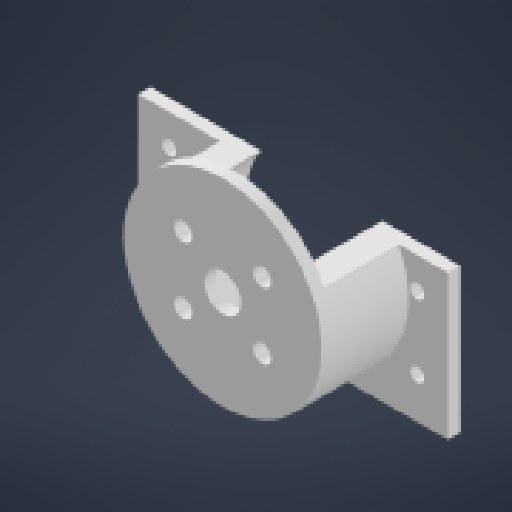
# Autodesk Inventor part: Rex Motor Bracket
Saved by Autodesk Inventor 2023 (Build 270158000, 158)
## iProperties
Created: 2022-12-08
Part Number: Rex Motor Bracket
Material: Generic
Document SubType Name: Modeling
Designer: Izack Waczko
Density: 1 g/cm^3
Appearance: Default
Author: Izack Waczko
Autodesk Inventor part; units mm, degrees
ref_plane "YZ Plane" through (0, 0, 0) normal (1, 0, 0) x (0, 1, 0)
ref_plane "XZ Plane" through (0, 0, 0) normal (0, 1, 0) x (-1, 0, 0)
sketch "Sketch1" plane through (0, 0, 0) normal (0, 0, 1) x (1, 0, 0)
  circle A0 centre (-15, 75) radius 1.7
  circle A1 centre (-15, 57.5) radius 1.7
  circle A2 centre (-75, 75) radius 1.7
  circle A3 centre (-75, 57.5) radius 1.7
  line L0 (-67.5, 62.5) -> (-67.5, 82.5)
  arc A4 (-67.5, 62.5) -> (-57.5, 52.5) centre (-57.5, 62.5) ccw
  line L1 (-32.5, 52.5) -> (-57.5, 52.5)
  arc A5 (-32.5, 52.5) -> (-22.5, 62.5) centre (-32.5, 62.5) ccw
  line L2 (-22.5, 82.5) -> (-22.5, 62.5)
  line L3 (-7.5, 82.5) -> (-22.5, 82.5)
  line L4 (-7.5, 62.5) -> (-7.5, 82.5)
  line L5 (-67.5, 82.5) -> (-82.5, 82.5)
  line L6 (-82.5, 82.5) -> (-82.5, -37.5)
  line L7 (-82.5, 52.5) -> (-57.5, 52.5)
  line L8 (-32.5, 52.5) -> (-7.5, 52.5)
  line L9 (-7.5, 52.5) -> (-7.5, 62.5)
  circle A6 centre (-41.087567, 72.129389) radius 17.98
  line L10 (-67.5, 82.5) -> (-55.775345, 82.5)
  line L11 (-22.5, 82.5) -> (-26.399789, 82.5)
  line L12 (-7.5, 52.5) -> (-82.5, 52.5)
  line L13 (-82.5, 52.5) -> (-82.5, 47.5)
  line L14 (-82.5, 47.5) -> (-7.5, 47.5)
  line L15 (-7.5, 47.5) -> (-7.5, 52.5)
  point P0 (0, 0)
  point P1 (-22.296102, 67.952867)
  dimension "d2" = 5
  constraints: 18 end point, 4 point on line, 3 perpendicular, 3 point on circle, 2 horizontal, 2 parallel, 1 other
  measures "d2" distance of L13.end L12.end
extrude "Extrusion1" add sketch "Sketch1" along normal blind 3 contours A4 L7 L6 L5 L0 | L0 L10 A6 L11 L2 A5 L1 A4 | L1 L8 L15 L14 L6 L7 | A5 L2 L3 L4 L9 L8
sketch "Sketch2" plane through (0, 0, 3) normal (0, 0, 1) x (1, 0, 0)
  circle A0 centre (-41.087567, 72.129389) radius 17.98
  line L0 (-55.775345, 82.5) -> (-82.5, 82.5)
  line L1 (-7.5, 82.5) -> (-26.399789, 82.5)
  circle A1 centre (-41.087567, 72.129389) radius 20.98
  point P0 (0, 0)
  point P1 (-59.325188, 82.5)
  point P2 (-22.849946, 82.5)
  dimension "d3" = 3
  constraints: 1 centre point
  measures "d3" radial gap between concentric circles of A0 A1
ref_plane "Work Plane1" through (-53.798179, 52.016597, 21) normal (0, 0, 1) x (0.817541, 0.5758704, 0)
extrude "Extrusion2" add sketch "Sketch2" along normal up to surface (18 mm away) contours A0 L1 A1 L0 picked at (-21.478975, 69.046328)
sketch "Sketch3" plane through (-41.087567, 72.129389, 21) normal (0, 0, 1) x (1, 0, 0)
  arc A0 (-18.237621, 10.370611) -> (18.237621, 10.370611) centre (0, 0) ccw
  circle A1 centre (0, 0) radius 4.485
  arc A2 (-14.687778, 10.370611) -> (14.687778, 10.370611) centre (0, 0) ccw construction
  line L0 (0, 0) -> (11.25, 0) construction
  line L1 (8, 0) -> (8, -8) construction
  line L2 (0, 0) -> (0, -11.25) construction
  circle A3 centre (8, -8) radius 2.2
  circle A4 centre (-8, -8) radius 2.2
  circle A5 centre (0, 0) radius 20.98
  circle A6 centre (8, 8) radius 2.2
  circle A7 centre (-8, 8) radius 2.2
  point P0 (41.087567, -72.129389)
  point P1 (18.237621, 10.370611)
  point P2 (-18.237621, 10.370611)
  dimension "d6" = 8
  dimension "d7" = 4.4
  dimension "d20" = 16
  dimension "d21" = 8
  constraints: 6 end point, 5 centre point, 3 symmetric about line, 2 coincident, 1 concentric, 1 horizontal, 1 perpendicular, 1 point on line, 1 vertical, 3 other
  measures "d6" distance of L1.start L1.end
  measures "d7" diameter of A3
  measures "d20" distance of A4.centre L1.end
  measures "d21" distance from line of L1 A0.centre
extrude "Extrusion3" add sketch "Sketch3" along normal blind 3
fillet "Fillet1" radius 5 4 edges at (-82.5, 82.5, 1.5) (-82.5, 47.5, 1.5) (-7.5, 47.5, 1.5) (-7.5, 82.5, 1.5)
fillet "Fillet2" radius 5 1 edges at (-41.0876, 51.1494, 3)
fillet "Fillet3" radius 5 1 edges at (-59.3252, 61.7588, 24)
sketch "Sketch4" plane through (0, 0, 3) normal (0, 0, 1) x (1, 0, 0)
  circle A0 centre (-15, 57.5) radius 1.7
  arc A1 (-15.134193, 73.305305) -> (-15.499481, 76.624967) centre (-15, 75) ccw
  circle A2 centre (-75, 75) radius 1.7
  circle A3 centre (-75, 57.5) radius 1.7
  circle A4 centre (-15, 57.5) radius 3.5
  circle A5 centre (-75, 57.5) radius 3.5
  circle A6 centre (-75, 75) radius 3.5
  circle A7 centre (-15, 75) radius 1.7
  circle A8 centre (-15, 75) radius 3.5
  point P0 (0, 0)
  dimension "d13" = 7
  dimension "d14" = 7
  dimension "d15" = 7
  dimension "d16" = 7
  constraints: 4 centre point, 4 coincident
  measures "d13" diameter of A4
  measures "d14" diameter of A5
  measures "d15" diameter of A6
  measures "d16" diameter of A8
extrude "Extrusion4" cut sketch "Sketch4" along normal blind 3
body "Solid1"
